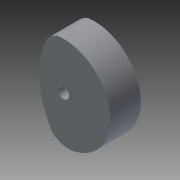
# Autodesk Inventor part: STAWPER 4.0
Saved by Autodesk Inventor 2015 (Build 190159000, 159)
## iProperties
Created: 2016-02-18
Part Number: STAWPER 4.0
Material: Generic
Document SubType Name: Modeling
Designer: JovinHo
Density: 1 g/cm^3
Appearance: Default
Author: JovinHo
Autodesk Inventor part; units mm, degrees
ref_plane "YZ Plane" through (0, 0, 0) normal (1, 0, 0) x (0, 1, 0)
ref_plane "XZ Plane" through (0, 0, 0) normal (0, 1, 0) x (-1, 0, 0)
ref_plane "XY Plane" through (0, 0, 0) normal (0, 0, 1) x (1, 0, 0)
sketch "Sketch1" plane through (0, 0, 0) normal (0, 0, 1) x (1, 0, 0)
  circle A0 centre (0, 0) radius 38.735
  line L0 (0, 0) -> (-20.2041, 0)
  arc A1 (-11.5296, 36.9793) -> (-20.2041, 0) centre (57.4407, 1.2934) ccw
  arc A2 (-20.2041, 0) -> (-5.8834, -38.2856) centre (57.1258, 7.104) ccw
  dimension "d0" = 77.47
  constraints: 6 point on circle, 3 centre point, 2 end point, 1 coincident, 1 horizontal
  measures "d0" diameter of A0
extrude "Extrusion1" add sketch "Sketch1" along normal blind 25.4 contours A0 A2 A1 picked at (-0.0151, -3.4014)
sketch "Sketch2" plane through (0, 0, 25.4) normal (0, 0, 1) x (1, 0, 0)
  arc A0 (-3.431, 38.8653) -> (-14.6706, 30.4652) centre (0.867, 21.3949) ccw
  arc A1 (-20.2041, 0) -> (-5.8834, -38.2856) centre (57.1258, 7.104) ccw projected
  arc A2 (-9.9035, -32.1064) -> (1.538, -38.2856) centre (0.2366, -27.013) ccw
  circle A3 centre (0, 0) radius 4.445
  dimension "d3" = 8.89
  constraints: 5 point on circle, 3 centre point, 1 coincident
  measures "d3" diameter of A3
extrude "Extrusion2" cut sketch "Sketch2" against normal through all fills toward (-9.9334, 35.8462) open curves A0
sketch "Sketch3" plane through (0, 0, 25.4) normal (0, 0, 1) x (1, 0, 0)
  arc A0 (-20.2041, 0) -> (-5.8834, -38.2856) centre (57.1258, 7.104) ccw projected
  arc A1 (-5.8834, -38.2856) -> (-4.9614, 38.4159) centre (0, 0) ccw projected
  arc A2 (-9.1874, -33.3056) -> (5.8834, -38.2856) centre (4.8247, -16.1952) ccw
  constraints: 4 point on circle, 1 centre point
extrude "Extrusion3" cut sketch "Sketch3" against normal through all
sketch "Sketch4" plane through (0, 0, 25.4) normal (0, 0, 1) x (1, 0, 0)
  circle A0 centre (0, 0) radius 4.572
  dimension "d9" = 9.144
  constraints: 1 centre point, 1 coincident
  measures "d9" diameter of A0
extrude "Extrusion4" cut sketch "Sketch4" against normal through all
body "Solid1"
